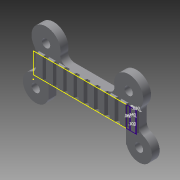
# Autodesk Inventor part: thinbumpyteeth
Saved by Autodesk Inventor 2013 SP2 (Build 170200200, 200)
## iProperties
Created: 2015-11-30
Part Number: thinbumpyteeth
Document SubType Name: Modeling
Designer: 2016ahoganso
Density: 1 g/cm^3
Material: Generic
Author: 2016ahoganso
Autodesk Inventor part; units mm, degrees
ref_plane "YZ Plane" through (0, 0, 0) normal (1, 0, 0) x (0, 1, 0)
ref_plane "XZ Plane" through (0, 0, 0) normal (0, 1, 0) x (-1, 0, 0)
ref_plane "XY Plane" through (0, 0, 0) normal (0, 0, 1) x (1, 0, 0)
sketch "Sketch1" plane through (0, 0, 0) normal (0, 0, 1) x (1, 0, 0)
  circle A0 centre (5.08, 17.272) radius 2.032
  arc A1 (11.178925, 13.47517) -> (0, 12.192) centre (5.08, 17.272) ccw
  line L0 (11.919764, 12.192) -> (38.880236, 12.192)
  circle A2 centre (45.72, 17.272) radius 2.032
  arc A3 (50.8, 12.192) -> (39.621075, 13.47517) centre (45.72, 17.272) ccw
  line L1 (0, 12.192) -> (0, 2.032)
  line L2 (50.8, 12.192) -> (50.8, 2.032)
  line L3 (11.919764, 12.192) -> (12.7, 12.192)
  line L4 (11.178925, 13.47517) -> (11.919764, 12.192)
  line L5 (38.880236, 12.192) -> (39.621075, 13.47517)
  line L6 (6.35, 2.032) -> (44.45, 2.032)
  circle A4 centre (0, -4.318) radius 2.032
  circle A5 centre (50.8, -4.318) radius 2.032
  arc A6 (0, 2.032) -> (6.016101, -6.35) centre (0, -4.318) ccw
  arc A7 (44.783899, -6.35) -> (50.8, 2.032) centre (50.8, -4.318) ccw
  line L7 (6.35, 2.032) -> (6.35, -6.096)
  line L8 (6.35, -6.096) -> (6.016101, -6.35)
  line L9 (44.45, 2.032) -> (44.234186, 2.032)
  line L10 (44.45, 2.032) -> (44.45, -6.096)
  line L11 (44.45, -6.096) -> (44.783899, -6.35)
  point P0 (10.16, 12.192)
  point P1 (10.16, 2.032)
  dimension "d28" = 11.91976
  dimension "d29" = 4.064
  dimension "d30" = 10.16
  dimension "d31" = 50.8
  dimension "d100" = 38.1
  constraints: 25 end point, 8 centre point, 8 point on circle, 4 coincident, 3 point on line, 2 other
  measures "d28" distance of L0.start L1.start
  measures "d29" diameter of A0
  measures "d30" distance between parallel lines of L0 L6
  measures "d31" distance between parallel lines of L2 L1
  measures "d100" distance of L6.start L6.end
extrude "Extrusion1" add sketch "Sketch1" along normal blind 6.35
fillet "Fillet1" radius 3.175 1 edges at (11.9198, 12.192, 3.175)
fillet "Fillet2" radius 3.175 1 edges at (11.1789, 13.4752, 3.175)
fillet "Fillet3" radius 3.175 1 edges at (38.8802, 12.192, 3.175)
fillet "Fillet4" radius 3.175 1 edges at (39.6101, 13.4929, 3.175)
fillet "Fillet5" radius 3.175 2 edges at (50.8, 12.192, 3.175) (50.8, 2.032, 3.175)
fillet "Fillet6" radius 3.175 2 edges at (0, 12.192, 3.175) (0, 2.032, 3.175)
sketch "Sketch2" plane through (0, 0, 6.35) normal (0, 0, 1) x (1, 0, 0)
  line L0 (15.262539, 12.192) -> (35.537461, 12.192)
  line L1 (44.45, 2.032) -> (6.35, 2.032)
  line L2 (0, 2.032) -> (50.8, 2.032)
  line L3 (50.8, 2.032) -> (50.8, 12.192)
  line L4 (50.8, 12.192) -> (0, 12.192)
  line L5 (0, 12.192) -> (0, 2.032)
  line L6 (0, 2.032) -> (2.54, 2.032)
  line L7 (2.54, 12.192) -> (0, 12.192)
  line L8 (0, 12.192) -> (0, 2.032)
  line L9 (2.54, 12.192) -> (5.08, 12.192)
  line L10 (5.08, 2.032) -> (2.54, 2.032)
  line L11 (5.08, 12.192) -> (7.62, 12.192)
  line L12 (7.62, 2.032) -> (5.08, 2.032)
  line L13 (7.62, 12.192) -> (10.16, 12.192)
  line L14 (10.16, 2.032) -> (7.62, 2.032)
  line L15 (10.16, 12.192) -> (12.7, 12.192)
  line L16 (12.7, 2.032) -> (10.16, 2.032)
  line L17 (12.7, 12.192) -> (15.24, 12.192)
  line L18 (15.24, 2.032) -> (12.7, 2.032)
  line L19 (15.262539, 12.192) -> (17.802539, 12.192)
  line L20 (17.802539, 2.032) -> (15.262539, 2.032)
  line L21 (17.802539, 12.192) -> (20.342539, 12.192)
  line L22 (20.342539, 2.032) -> (17.802539, 2.032)
  line L23 (20.342539, 12.192) -> (22.882539, 12.192)
  line L24 (22.882539, 2.032) -> (20.342539, 2.032)
  line L25 (22.882539, 12.192) -> (25.422539, 12.192)
  line L26 (25.422539, 2.032) -> (22.882539, 2.032)
  line L27 (25.422539, 12.192) -> (27.962539, 12.192)
  line L28 (27.962539, 2.032) -> (25.422539, 2.032)
  line L29 (27.962539, 12.192) -> (30.502539, 12.192)
  line L30 (30.502539, 2.032) -> (27.962539, 2.032)
  line L31 (30.502539, 12.192) -> (33.042539, 12.192)
  line L32 (33.042539, 2.032) -> (30.502539, 2.032)
  line L33 (33.042539, 12.192) -> (35.582539, 12.192)
  line L34 (35.582539, 2.032) -> (33.042539, 2.032)
  line L35 (35.537461, 12.192) -> (38.077461, 12.192)
  line L36 (38.077461, 2.032) -> (35.537461, 2.032)
  line L37 (38.077461, 12.192) -> (40.617461, 12.192)
  line L38 (40.617461, 2.032) -> (38.077461, 2.032)
  line L39 (40.617461, 12.192) -> (43.157461, 12.192)
  line L40 (43.157461, 2.032) -> (40.617461, 2.032)
  line L41 (43.157461, 12.192) -> (45.697461, 12.192)
  line L42 (45.697461, 2.032) -> (43.157461, 2.032)
  line L43 (45.697461, 12.192) -> (48.237461, 12.192)
  line L44 (48.237461, 2.032) -> (45.697461, 2.032)
  line L45 (48.237461, 12.192) -> (50.777461, 12.192)
  line L46 (50.777461, 2.032) -> (48.237461, 2.032)
  line L47 (33.042539, 12.192) -> (35.582539, 12.192)
  line L48 (35.582539, 2.032) -> (33.042539, 2.032)
  line L49 (50.777461, 12.192) -> (50.777461, 2.032)
  line L50 (48.237461, 12.192) -> (50.777461, 12.192)
  line L51 (50.777461, 2.032) -> (48.237461, 2.032)
  line L52 (50.777461, 2.032) -> (50.777461, 12.192)
  line L53 (50.777461, 2.032) -> (50.777461, 12.192)
  line L54 (45.697461, 12.192) -> (48.237461, 12.192)
  line L55 (48.237461, 2.032) -> (45.697461, 2.032)
  line L56 (43.157461, 12.192) -> (45.697461, 12.192)
  line L57 (45.697461, 2.032) -> (43.157461, 2.032)
  line L58 (40.617461, 12.192) -> (43.157461, 12.192)
  line L59 (43.157461, 2.032) -> (40.617461, 2.032)
  line L60 (38.077461, 12.192) -> (40.617461, 12.192)
  line L61 (40.617461, 2.032) -> (38.077461, 2.032)
  line L62 (35.537461, 12.192) -> (38.077461, 12.192)
  line L63 (38.077461, 2.032) -> (35.537461, 2.032)
  point P0 (6.096, 2.032)
  point P1 (44.704, 2.032)
  point P2 (0, 0)
  dimension "d43" = 50.8
  constraints: 124 end point, 29 parallel, 28 horizontal, 4 point on line, 2 perpendicular
  measures "d43" distance of L2.start L2.end
extrude "Extrusion2" add sketch "Sketch2" along normal blind 1.2446
sketch "Sketch3" plane through (0, 0, 7.5946) normal (0, 0, 1) x (1, 0, 0)
  line L0 (0, 2.032) -> (0, 12.192) projected
  line L1 (50.8, 2.032) -> (0, 2.032) projected
  line L2 (50.8, 12.192) -> (50.8, 2.032) projected
  line L3 (0, 12.192) -> (50.8, 12.192) projected
  line L4 (50.8, 12.192) -> (47.244, 12.192)
  line L5 (47.244, 12.192) -> (47.244, 2.032)
  line L6 (47.244, 2.032) -> (50.8, 2.032)
  line L7 (50.8, 2.032) -> (50.8, 12.192)
  line L8 (47.244, 12.192) -> (45.72, 12.192)
  line L9 (45.72, 12.192) -> (45.72, 2.032)
  line L10 (45.72, 2.032) -> (47.244, 2.032)
  line L11 (47.244, 2.032) -> (47.244, 12.192)
  line L12 (50.8, 12.192) -> (50.292, 12.192)
  line L13 (50.292, 12.192) -> (47.752, 12.192)
  line L14 (47.752, 12.192) -> (47.752, 2.032)
  line L15 (47.752, 2.032) -> (50.292, 2.032)
  line L16 (50.292, 2.032) -> (50.292, 12.192)
  point P0 (0, 0)
  dimension "d71" = 3.556
  dimension "d72" = 1.524
  dimension "d73" = 0.508
  dimension "d74" = 2.54
  constraints: 26 end point, 6 parallel, 4 point on line, 3 horizontal, 3 perpendicular
  measures "d71" distance between parallel lines of L5 L7
  measures "d72" distance between parallel lines of L9 L11
  measures "d73" distance of L2.start L12.end
  measures "d74" distance between parallel lines of L14 L16
sketch "Sketch4" plane through (0, 12.192, 6.35) normal (0, 1, 0) x (1, 0, 0)
  line L0 (0, -1.2446) -> (50.8, -1.2446)
  line L1 (50.8, 0) -> (50.8, -1.2446)
  line L2 (35.537461, 0) -> (50.8, 0)
  line L3 (50.8, 0) -> (50.292, 0)
  line L4 (50.292, 0) -> (50.292, -1.2446)
  line L5 (50.292, -1.2446) -> (50.8, 0)
  point P0 (0, 6.35)
  dimension "d75" = 0.508
  constraints: 6 end point, 2 point on line, 1 perpendicular
  measures "d75" distance of L1.start L3.end
extrude "Extrusion3" cut sketch "Sketch4" against normal blind 25.4 contours L5 L1 L0
sketch "Sketch5" plane through (6.096, 2.032, 0) normal (0, -1, 0) x (1, 0, 0)
  line L0 (44.196, 7.5946) -> (-6.096, 7.5946)
  line L1 (-6.096, 6.35) -> (-6.096, 7.5946)
  line L2 (44.704, 6.35) -> (-6.096, 6.35)
  line L3 (44.704, 6.35) -> (41.148, 6.35)
  line L4 (41.656, 7.5946) -> (41.148, 6.35)
  line L5 (41.148, 6.35) -> (39.624, 6.35)
  line L6 (39.624, 6.35) -> (39.116, 7.5946)
  line L7 (44.196, 7.5946) -> (41.656, 7.5946)
  line L8 (36.576, 7.5946) -> (36.068, 6.35)
  line L9 (36.068, 6.35) -> (34.544, 6.35)
  line L10 (34.544, 6.35) -> (34.036, 7.5946)
  line L11 (39.116, 7.5946) -> (36.576, 7.5946)
  line L12 (31.496, 7.5946) -> (30.988, 6.35)
  line L13 (30.988, 6.35) -> (29.464, 6.35)
  line L14 (29.464, 6.35) -> (28.956, 7.5946)
  line L15 (34.036, 7.5946) -> (31.496, 7.5946)
  line L16 (26.416, 7.5946) -> (25.908, 6.35)
  line L17 (25.908, 6.35) -> (24.384, 6.35)
  line L18 (24.384, 6.35) -> (23.876, 7.5946)
  line L19 (28.956, 7.5946) -> (26.416, 7.5946)
  line L20 (21.336, 7.5946) -> (20.828, 6.35)
  line L21 (20.828, 6.35) -> (19.304, 6.35)
  line L22 (19.304, 6.35) -> (18.796, 7.5946)
  line L23 (23.876, 7.5946) -> (21.336, 7.5946)
  line L24 (16.256, 7.5946) -> (15.748, 6.35)
  line L25 (15.748, 6.35) -> (14.224, 6.35)
  line L26 (14.224, 6.35) -> (13.716, 7.5946)
  line L27 (18.796, 7.5946) -> (16.256, 7.5946)
  line L28 (11.176, 7.5946) -> (10.668, 6.35)
  line L29 (10.668, 6.35) -> (9.144, 6.35)
  line L30 (9.144, 6.35) -> (8.636, 7.5946)
  line L31 (13.716, 7.5946) -> (11.176, 7.5946)
  line L32 (6.096, 7.5946) -> (5.588, 6.35)
  line L33 (5.588, 6.35) -> (4.064, 6.35)
  line L34 (4.064, 6.35) -> (3.556, 7.5946)
  line L35 (8.636, 7.5946) -> (6.096, 7.5946)
  line L36 (1.016, 7.5946) -> (0.508, 6.35)
  line L37 (0.508, 6.35) -> (-1.016, 6.35)
  line L38 (-1.016, 6.35) -> (-1.524, 7.5946)
  line L39 (3.556, 7.5946) -> (1.016, 7.5946)
  line L40 (-4.064, 7.5946) -> (-4.572, 6.35)
  line L41 (-4.572, 6.35) -> (-6.096, 6.35)
  line L42 (-1.524, 7.5946) -> (-4.064, 7.5946)
  line L43 (-6.096, 6.35) -> (-6.096, 7.5946)
  line L44 (-4.064, 7.5946) -> (-6.096, 7.5946)
  line L45 (-1.524, 7.5946) -> (1.016, 7.5946)
  line L46 (3.556, 7.5946) -> (6.388906, 7.5946)
  line L47 (8.636, 7.5946) -> (11.600674, 7.5946)
  line L48 (13.716, 7.5946) -> (41.656, 7.5946)
  line L49 (3.556, 7.5946) -> (6.096, 7.5946)
  line L50 (8.636, 7.5946) -> (11.176, 7.5946)
  line L51 (13.716, 7.5946) -> (16.256, 7.5946)
  line L52 (18.796, 7.5946) -> (21.336, 7.5946)
  line L53 (23.876, 7.5946) -> (26.416, 7.5946)
  line L54 (28.956, 7.5946) -> (31.496, 7.5946)
  line L55 (34.036, 7.5946) -> (36.576, 7.5946)
  line L56 (39.116, 7.5946) -> (41.656, 7.5946)
  point P0 (38.608, 6.35)
  point P1 (-6.096, 0)
  dimension "d78" = 3.556
  dimension "d80" = 1.524
  dimension "d82" = 1.524
  dimension "d83" = 1.524
  dimension "d84" = 1.524
  dimension "d85" = 1.524
  dimension "d86" = 1.524
  dimension "d87" = 1.524
  dimension "d88" = 1.524
  dimension "d89" = 1.524
  dimension "d90" = 1.524
  constraints: 108 end point, 12 collinear, 6 point on line, 1 perpendicular
  measures "d78" distance of L2.start L3.end
  measures "d80" distance of L3.end L5.end
  measures "d82" distance of L8.end L9.end
  measures "d83" distance of L12.end L13.end
  measures "d84" distance of L16.end L17.end
  measures "d85" distance of L20.end L21.end
  measures "d86" distance of L24.end L25.end
  measures "d87" distance of L28.end L29.end
  measures "d88" distance of L32.end L33.end
  measures "d89" distance of L36.end L37.end
  measures "d90" distance of L40.end L1.start
sketch "Sketch5 outline for Extrusion4" plane through (6.096, 2.032, 0) normal (0, -1, 0) x (1, 0, 0)
  line L0 (39.624, 6.35) -> (41.148, 6.35)
  line L1 (39.116, 7.5946) -> (39.624, 6.35)
  line L2 (41.656, 7.5946) -> (39.116, 7.5946)
  line L3 (41.148, 6.35) -> (41.656, 7.5946)
  line L4 (-4.064, 7.5946) -> (-6.096, 7.5946)
  line L5 (-4.572, 6.35) -> (-4.064, 7.5946)
  line L6 (-6.096, 6.35) -> (-4.572, 6.35)
  line L7 (-6.096, 7.5946) -> (-6.096, 6.35)
  line L8 (20.828, 6.35) -> (21.336, 7.5946)
  line L9 (19.304, 6.35) -> (20.828, 6.35)
  line L10 (18.796, 7.5946) -> (19.304, 6.35)
  line L11 (21.336, 7.5946) -> (18.796, 7.5946)
  line L12 (30.988, 6.35) -> (31.496, 7.5946)
  line L13 (29.464, 6.35) -> (30.988, 6.35)
  line L14 (28.956, 7.5946) -> (29.464, 6.35)
  line L15 (31.496, 7.5946) -> (28.956, 7.5946)
  line L16 (5.588, 6.35) -> (6.096, 7.5946)
  line L17 (4.064, 6.35) -> (5.588, 6.35)
  line L18 (3.556, 7.5946) -> (4.064, 6.35)
  line L19 (6.096, 7.5946) -> (3.556, 7.5946)
  line L20 (10.668, 6.35) -> (11.176, 7.5946)
  line L21 (9.144, 6.35) -> (10.668, 6.35)
  line L22 (8.636, 7.5946) -> (9.144, 6.35)
  line L23 (11.176, 7.5946) -> (8.636, 7.5946)
  line L24 (16.256, 7.5946) -> (13.716, 7.5946)
  line L25 (15.748, 6.35) -> (16.256, 7.5946)
  line L26 (14.224, 6.35) -> (15.748, 6.35)
  line L27 (13.716, 7.5946) -> (14.224, 6.35)
  line L28 (0.508, 6.35) -> (1.016, 7.5946)
  line L29 (-1.016, 6.35) -> (0.508, 6.35)
  line L30 (-1.524, 7.5946) -> (-1.016, 6.35)
  line L31 (1.016, 7.5946) -> (-1.524, 7.5946)
  line L32 (25.908, 6.35) -> (26.416, 7.5946)
  line L33 (24.384, 6.35) -> (25.908, 6.35)
  line L34 (23.876, 7.5946) -> (24.384, 6.35)
  line L35 (26.416, 7.5946) -> (23.876, 7.5946)
  line L36 (36.068, 6.35) -> (36.576, 7.5946)
  line L37 (34.544, 6.35) -> (36.068, 6.35)
  line L38 (34.036, 7.5946) -> (34.544, 6.35)
  line L39 (36.576, 7.5946) -> (34.036, 7.5946)
extrude "Extrusion4" cut sketch "Sketch5 outline for Extrusion4" against normal blind 25.4
sketch "Sketch9" plane through (0, 0, 0) normal (0, 0, -1) x (-1, 0, 0)
  arc A0 (-52.916667, 1.668837) -> (-44.783899, -6.35) centre (-50.8, -4.318) ccw
  line L0 (-44.45, -6.096) -> (-44.783899, -6.35)
  line L1 (-44.45, 2.032) -> (-44.45, -6.096)
  line L2 (-6.35, 2.032) -> (-44.45, 2.032)
  line L3 (-6.35, -6.096) -> (-6.35, 2.032)
  line L4 (-6.016101, -6.35) -> (-6.35, -6.096)
  arc A1 (-6.016101, -6.35) -> (2.116667, 1.668837) centre (0, -4.318) ccw
  arc A2 (0, 4.662256) -> (2.116667, 1.668837) centre (3.175, 4.662256) ccw
  line L5 (0, 11.013558) -> (0, 4.662256)
  arc A3 (0.644919, 12.931712) -> (0, 11.013558) centre (3.175, 11.013558) ccw
  arc A4 (0.644919, 12.931712) -> (-12.141685, 15.950865) centre (-5.08, 17.272) ccw
  arc A5 (-15.262539, 12.192) -> (-12.141685, 15.950865) centre (-15.262539, 15.367) ccw
  line L6 (-35.537461, 12.192) -> (-15.262539, 12.192)
  arc A6 (-38.658315, 15.950865) -> (-35.537461, 12.192) centre (-35.537461, 15.367) ccw
  arc A7 (-38.658315, 15.950865) -> (-51.444919, 12.931712) centre (-45.72, 17.272) ccw
  arc A8 (-50.8, 11.013558) -> (-51.444919, 12.931712) centre (-53.975, 11.013558) ccw
  line L7 (-50.8, 4.662256) -> (-50.8, 11.013558)
  arc A9 (-52.916667, 1.668837) -> (-50.8, 4.662256) centre (-53.975, 4.662256) ccw
  circle A10 centre (-50.8, -4.318) radius 2.032
  circle A11 centre (0, -4.318) radius 2.032
  circle A12 centre (-45.72, 17.272) radius 2.032
  circle A13 centre (-5.08, 17.272) radius 2.032
  point P0 (0, 0)
extrude "Extrusion6" cut sketch "Sketch9" against normal blind 2.54
body "Solid1"
